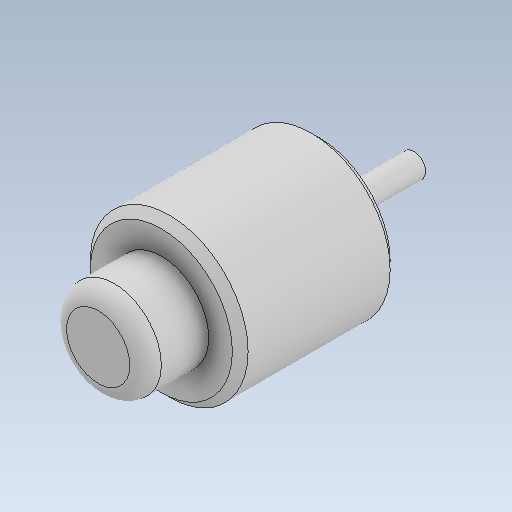
# Autodesk Inventor part: DC motor_CPY1
Saved by Autodesk Inventor 2021 (Build 250183000, 183)
## iProperties
Created: 2021-06-27
Part Number: DC motor_CPY1
Material: Generic
Document SubType Name: Modeling
Designer: Manojgouda K R
Density: 1 g/cm^3
Appearance: Default
Author: Manojgouda K R
Autodesk Inventor part; units mm, degrees
ref_plane "YZ Plane" through (0, 0, 0) normal (1, 0, 0) x (0, 1, 0)
ref_plane "XZ Plane" through (0, 0, 0) normal (0, 1, 0) x (-1, 0, 0)
ref_plane "XY Plane" through (0, 0, 0) normal (0, 0, 1) x (1, 0, 0)
sketch "Sketch1" plane through (0, 0, 0) normal (0, 0, 1) x (1, 0, 0)
  circle A0 centre (0, 0) radius 2.5
  dimension "d0" = 5
  constraints: 1 centre point, 1 coincident
  measures "d0" diameter of A0
extrude "Extrusion1" add sketch "Sketch1" along normal blind 5
chamfer "Chamfer1" distance 0.25 angle 45 2 edges at (-2.5, 0, 5) (-2.5, 0, 0)
sketch "Sketch2" plane through (0, 0, 5) normal (0, 0, 1) x (1, 0, 0)
  circle A0 centre (0, 0) radius 1.5
  dimension "d12" = 3
  constraints: 1 centre point, 1 coincident
  measures "d12" diameter of A0
extrude "Extrusion2" add sketch "Sketch2" along normal blind 2
fillet "Fillet1" radius 0.5 1 edges at (-1.5, 0, 7)
sketch "Sketch3" plane through (0, 0, 0) normal (0, 0, -1) x (-1, 0, 0)
  circle A0 centre (0, 0) radius 0.375
  dimension "d9" = 0.75
  constraints: 1 centre point, 1 coincident
  measures "d9" diameter of A0
extrude "Extrusion3" add sketch "Sketch3" along normal blind 3
body "Solid1"
